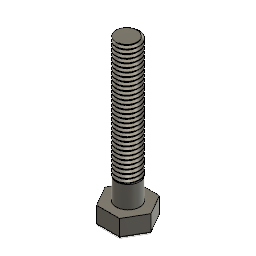
17part (Autodesk Fusion 360 design; units mm, degrees)
Autodesk Fusion 360 part; units mm, degrees
sketch "Sketch1" plane through (0, 0, 0) normal (0, 1, 0) x (1, 0, 0)
  circle A0 centre (0, 0) radius 3
  line L0 (-2.8868, 5) -> (-5.7735, 0)
  line L1 (-5.7735, 0) -> (-2.8868, -5)
  line L2 (-2.8868, -5) -> (2.8868, -5)
  line L3 (2.8868, -5) -> (5.7735, 0)
  line L4 (5.7735, 0) -> (2.8868, 5)
  line L5 (2.8868, 5) -> (-2.8868, 5)
  dimension "d1" = 6
  dimension "d2" = 5
  constraint coincident A0.centre origin
  constraint horizontal L5
  measures "d1" diameter of A0
  measures "d2" distance of A0.centre L5
extrude "Extrude1" add sketch "Sketch1" along normal blind 40 contours A0
extrude "Extrude2" add sketch "Sketch1" along normal blind 4.5
fillet "Fillet1" radius 0.5 1 faces at (0.9623, 0, -1.6667)
thread "Thread1" "ISO Metric profile 6.0 M6x1 6g" major diameter 5.884 minor diameter 4.7435 pitch 1 angle 60 modelled right hand crest width 0.125 on face at (2.9851, 16.3333, 0.2987) from (0, 10, 0) to (0, 40, 0) crest through (2.942, 4.4375, 0)
